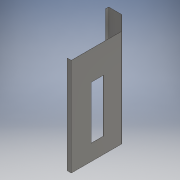
# Autodesk Inventor part: Cover Back
Saved by Autodesk Inventor 2018 (Build 220112000, 112)
## iProperties
Created: 2018-08-07
Part Number: Cover Back
Material: Stainless Steel
Document SubType Name: Modeling
Designer: P301319
Density: 8 g/cm^3
Appearance: Stainless - Brushed
Author: P301319
Autodesk Inventor part; units mm, degrees
ref_plane "YZ Plane" through (0, 0, 0) normal (1, 0, 0) x (0, 1, 0)
ref_plane "XZ Plane" through (0, 0, 0) normal (0, 1, 0) x (-1, 0, 0)
ref_plane "XY Plane" through (0, 0, 0) normal (0, 0, 1) x (1, 0, 0)
sketch "Sketch1" plane through (0, 0, 0) normal (0, 0, 1) x (1, 0, 0)
  line L0 (-340, 800) -> (-180, 800)
  line L1 (-180, 800) -> (0, 620)
  line L2 (-180, 800) -> (122.4624, 800) construction
  line L3 (0, 0) -> (0, 620)
  line L4 (0, 0) -> (-50, 0)
  line L5 (-340, 800) -> (-340, 760)
  line L6 (-50, 1.6) -> (-1.6, 1.6)
  line L7 (-1.6, 1.6) -> (-1.6, 619.3373)
  line L8 (-1.6, 619.3373) -> (-180.6627, 798.4)
  line L9 (-180.6627, 798.4) -> (-338.4, 798.4)
  line L10 (-338.4, 798.4) -> (-338.4, 760)
  line L11 (-340, 760) -> (-338.4, 760)
  line L12 (-50, 1.6) -> (-50, 0)
  dimension "d0" = 160
  dimension "d1" = 45
  dimension "d2" = 800
  dimension "d4" = 50
  dimension "d15" = 180
  dimension "d16" = 40
  dimension "d17" = 1.6
  constraints: 26 end point, 4 horizontal, 3 vertical, 4 other
  measures "d0" distance of L0.start L0.end
  measures "d1" angle of L1 L2
  measures "d2" distance from line of L3.start L0
  measures "d4" distance of L3.start L4.end
  measures "d15" distance from line of L3 L0.end
  measures "d16" distance of L0.start L5.end
  measures "d17" distance between parallel lines of L0 L9
extrude "Extrusion1" add sketch "Sketch1" along normal blind 1200
sketch "Sketch2" plane through (0, 0, 0) normal (1, 0, 0) x (0, 0, -1)
  line L0 (-195, 320) -> (-845, 320) construction
  line L1 (-845, 395) -> (-195, 395)
  line L2 (-195, 395) -> (-195, 245)
  line L3 (-195, 245) -> (-845, 245)
  line L4 (-845, 245) -> (-845, 395)
  point P0 (0, 0)
  dimension "d8" = 195
  dimension "d9" = 320
  dimension "d10" = 650
  dimension "d11" = 650
  dimension "d12" = 150
  constraints: 10 end point, 2 horizontal, 2 parallel, 1 midpoint, 1 perpendicular
  measures "d8" horizontal distance of point (0, 0) L0.start
  measures "d9" distance from line of point (0, 0) L0
  measures "d10" distance of L0.end L0.start
  measures "d11" distance of L2.end L3.end
  measures "d12" distance of L1.end L2.end
extrude "Extrusion2" cut sketch "Sketch2" against normal blind 1200
body "Solid1"
